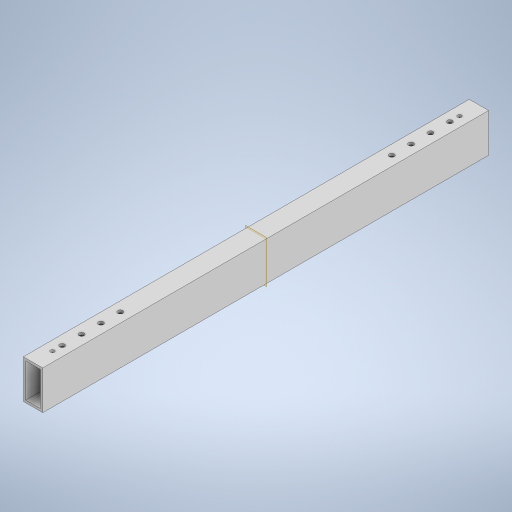
# Autodesk Inventor part: Drivetrain-Front-Back-Extrusions
Saved by Autodesk Inventor 2024.2 (Build 282272000, 272)
## iProperties
Created: 2024-01-04
Part Number: Drivetrain-Front-Back-Extrusions
Material: Generic
Document SubType Name: Modeling
Designer: rohan
Density: 1 g/cm^3
Appearance: Default
Author: rohan
Autodesk Inventor part; units mm, degrees
ref_plane "YZ Plane" through (0, 0, 0) normal (1, 0, 0) x (0, 1, 0)
ref_plane "XZ Plane" through (0, 0, 0) normal (0, 1, 0) x (-1, 0, 0)
ref_plane "XY Plane" through (0, 0, 0) normal (0, 0, 1) x (1, 0, 0)
sketch "Sketch1" plane through (0, 0, 0) normal (0, 0, 1) x (1, 0, 0)
  line L0 (-12.7, -25.4) -> (12.7, -25.4)
  line L1 (12.7, -25.4) -> (12.7, 25.4)
  line L2 (12.7, 25.4) -> (-12.7, 25.4)
  line L3 (-12.7, 25.4) -> (-12.7, -25.4)
  line L4 (-12.7, -25.4) -> (12.7, 25.4) construction
  line L5 (12.7, -25.4) -> (-12.7, 25.4) construction
  line L6 (-9.525, -22.225) -> (9.525, -22.225)
  line L7 (9.525, -22.225) -> (9.525, 22.225)
  line L8 (9.525, 22.225) -> (-9.525, 22.225)
  line L9 (-9.525, 22.225) -> (-9.525, -22.225)
  point P0 (0, 0)
  dimension "d0" = 25.4
  dimension "d1" = 50.8
  dimension "d2" = 3.175
  constraints: 20 end point, 4 parallel, 2 midpoint, 2 perpendicular, 1 horizontal, 3 other
  measures "d0" distance of L2.end L1.end
  measures "d1" distance of L1.end L0.end
  measures "d2" distance between parallel lines of L3 L9
extrude "Extrusion1" add sketch "Sketch1" along normal blind 584.2
sketch "Sketch2" plane through (-12.7, 25.4, 0) normal (0, 1, 0) x (1, 0, 0)
  circle A0 centre (12.7, -25.4) radius 2.5527
  circle A1 centre (12.7, -38.1) radius 3.2639
  line L0 (25.4, 0) -> (25.4, -584.2) projected
  circle A2 centre (12.7, -63.5) radius 3.2639
  circle A3 centre (12.7, -88.9) radius 3.2639
  circle A4 centre (12.7, -114.3) radius 3.2639
  point P0 (12.7, 0)
  dimension "d5" = 5.1054
  dimension "d6" = 25.4
  dimension "d7" = 6.5278
  dimension "d8" = 38.1
  dimension "d11" = 25.4
  constraints: 5 centre point, 1 vertical, 6 other
  measures "d5" diameter of A0
  measures "d6" distance of A0.centre point (12.7, 0)
  measures "d7" diameter of A1
  measures "d8" distance of A1.centre point (12.7, 0)
  measures "d11" distance of A1.centre A2.centre
extrude "Extrusion2" cut sketch "Sketch2" against normal blind 33.3375
ref_plane "Work Plane1" through (0, 0, 292.1) normal (0, 0, 1) x (1, 0, 0)
mirror "Mirror1" about plane through (0, 0, 292.1) normal (0, 0, 1) of "Extrusion2"
equation "\"d3\" = Length"
equation "\"Length\" = 584.2"
body "Solid1"
